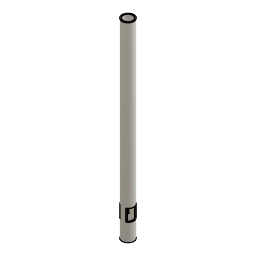
Body (Autodesk Fusion 360 archive; units mm, degrees)
design "Pipe"
part number: 2026-04-14-16-00-10-104
Autodesk Fusion 360 part; units mm, degrees
sketch "Sketch1" plane through (0, 0, 0) normal (0, 1, 0) x (1, 0, 0)
  circle A0 centre (0, 0) radius 5
  circle A1 centre (0, 0) radius 4
  dimension "d1" = 10
  dimension "d2" = 8
  constraint coincident A0.centre A1.centre
  measures "d1" diameter of A0
  measures "d2" diameter of A1
extrude "Extrude1" add sketch "Sketch1" along normal blind 160
sketch "Sketch2" plane through (0, 0, 0) normal (0, 0, 1) x (1, 0, 0)
  line L0 (-5, 0) -> (5, 0)
  line L1 (5, 0) -> (5, 15)
  line L2 (5, 15) -> (-5, 15)
  line L3 (-5, 15) -> (-5, 0)
  line L4 (-5, 15) -> (5, 15)
  line L5 (5, 15) -> (5, 25)
  line L6 (5, 25) -> (-5, 25)
  line L7 (-5, 25) -> (-5, 15)
  line L8 (-5, 25) -> (-2.5, 25)
  line L9 (-2.5, 25) -> (-2.5, 15)
  line L10 (-2.5, 15) -> (-5, 15)
  line L11 (-5, 15) -> (-5, 25)
  line L12 (5, 15) -> (2.5, 15)
  line L13 (2.5, 15) -> (2.5, 25)
  line L14 (2.5, 25) -> (5, 25)
  line L15 (5, 25) -> (5, 15)
  dimension "d5" = 10
  dimension "d6" = 15
  dimension "d7" = 10
  dimension "d8" = 10
  dimension "d9" = 2.5
  dimension "d10" = 10
  dimension "d11" = 2.5
  dimension "d12" = 10
  constraint horizontal L0
  constraint vertical L1
  constraint horizontal L2
  constraint vertical L3
  constraint horizontal L4
  constraint vertical L5
  constraint horizontal L6
  constraint vertical L7
  constraint horizontal L8
  constraint vertical L9
  constraint horizontal L10
  constraint vertical L11
  constraint horizontal L12
  constraint vertical L13
  constraint horizontal L14
  constraint vertical L15
  measures "d5" distance of L0.start L0.end
  measures "d6" distance of L0.start L2.end
  measures "d7" distance of L2.end L1.end
  measures "d8" distance of L2.end L6.end
  measures "d9" distance of L6.end L8.end
  measures "d10" distance of L6.end L2.end
  measures "d11" distance of L1.end L12.end
  measures "d12" distance of L1.end L5.end
extrude "Extrude2" cut sketch "Sketch2" along normal mid plane 20 contours L2 L4 L6 L7 L8 L9 L10 L11 | L2 L4 L5 L6 L12 L13 L14 L15
equation "d2 = d1 - 2 mm"
equation "d5 = d1"
equation "d7 = d1"
equation "d9 = d1 / 4"
equation "d10 = d1"
equation "d11 = d1 / 4"
equation "d12 = d1"
equation "d13 = d1"
named bodies: "Pipe"
